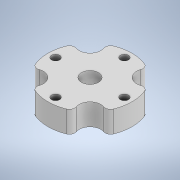
# Autodesk Inventor part: lüfter_flansch
Saved by Autodesk Inventor 2022 (Build 260153000, 153)
## iProperties
Created: 2022-01-28
Part Number: lüfter_flansch
Material: Generisch
Document SubType Name: Modeling
Designer: ga76xid
Density: 1 g/cm^3
Appearance: Vorgabe
Author: ga76xid
Autodesk Inventor part; units mm, degrees
ref_plane "XZ Plane" through (0, 0, 0) normal (0, 1, 0) x (-1, 0, 0)
sketch "Skizze1" plane through (0, 0, 0) normal (0, 1, 0) x (-1, 0, 0)
  circle A0 centre (0, 0) radius 3.14
  circle A1 centre (0, 0) radius 12.7
  circle A2 centre (0, 0) radius 15.5
  circle A3 centre (0, 12.7) radius 1.5
  circle A4 centre (12.7, 0) radius 1.5
  circle A5 centre (0, -12.7) radius 1.5
  circle A6 centre (-12.7, 0) radius 1.5
  dimension "d0" = 6.28
  dimension "d1" = 25.4
  dimension "d2" = 31
  dimension "d3" = 3
  dimension "d4" = 3
  dimension "d5" = 3
  dimension "d6" = 3
  constraints: 7 centre point, 4 point on circle, 3 coincident
  measures "d0" diameter of A0
  measures "d1" diameter of A1
  measures "d2" diameter of A2
  measures "d3" diameter of A3
  measures "d4" diameter of A4
  measures "d5" diameter of A5
  measures "d6" diameter of A6
extrude "Extrusion1" add sketch "Skizze1" along normal blind 8 contours A4 A1 A5 A6 A3 | A2
ref_plane "Arbeitsebene3" through (-10.9602, 0, 10.9602) normal (-0.7071, 0, 0.7071) x (0, -1, 0)
ref_plane "Arbeitsebene2" through (0, 0, 0) normal (-0.7071, 0, 0.7071) x (0, -1, 0)
sketch "Skizze2" plane through (-10.9602, 0, 10.9602) normal (-0.7071, 0, 0.7071) x (0, -1, 0)
  circle A0 centre (-4, 0) radius 1.475
  line L0 (0, 15.5) -> (0, -15.5) projected
  point P0 (0, 0)
  dimension "d9" = 2.95
  dimension "d10" = 4
  constraints: 1 centre point
  measures "d9" diameter of A0
  measures "d10" distance from line of L0 A0.centre
extrude "Extrusion2" cut sketch "Skizze2" against normal blind 16
sketch "Skizze3" plane through (0, 0, 0) normal (0, -1, 0) x (1, 0, 0)
  circle A0 centre (0, 0) radius 15.5 projected
  arc A1 (-11.9125, 6.8258) -> (-6.8258, 11.9125) centre (-10.6066, 10.6066) ccw
  line L0 (0, 0) -> (-15.0003, 15.0003) construction
  line L1 (0, 0) -> (0, 6.573) construction
  arc A2 (-14.4271, 5.6666) -> (-5.6666, 14.4271) centre (0, 0) ccw
  arc A3 (-11.9125, 6.8258) -> (-14.4271, 5.6666) centre (-12.5655, 4.9354) ccw
  arc A4 (-5.6666, 14.4271) -> (-6.8258, 11.9125) centre (-4.9354, 12.5655) ccw
  point P0 (-5.6666, 14.4271)
  point P1 (-14.4271, 5.6666)
  dimension "d13" = 8
  dimension "d14" = 45
  dimension "d15" = 2
  dimension "d18" = 15
  constraints: 8 point on circle, 4 centre point, 4 end point, 4 tangent, 2 equal radius, 1 coincident, 1 point on line, 1 vertical
  measures "d13" diameter of A1
  measures "d14" angle of L1 L0
  measures "d15" radius of A3
  measures "d18" distance of point (0, 0) A1.centre
extrude "Extrusion3" cut sketch "Skizze3" against normal blind 16 contours A4 A1 A3 A0 picked at (-11.6232, 8.691)
pattern_circular "Runde Anordnung1" count 4 over 360 about axis through (0, 0, 0) along (0, 1, 0) of "Extrusion3"
